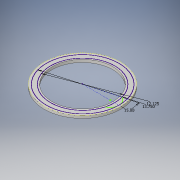
# Autodesk Inventor part: DiskCam
Saved by Autodesk Inventor 2016 (Build 200138000, 138)
## iProperties
Created: 2015-07-20
Part Number: DiskCam
Material: PC/ABS Plastic
Document SubType Name: Modeling
Designer: steele
Density: 0.357273 g/cm^3
Appearance: Smooth - White
Mass: 179.331 g
Surface Area: 1053.95 cm^2
Volume: 501.944 cm^3
Author: steele
Autodesk Inventor part; units mm, degrees
ref_plane "YZ Plane" through (0, 0, 0) normal (1, 0, 0) x (0, 1, 0)
ref_plane "XZ Plane" through (0, 0, 0) normal (0, 1, 0) x (-1, 0, 0)
ref_plane "XY Plane" through (0, 0, 0) normal (0, 0, 1) x (1, 0, 0)
sketch "Sketch1" plane through (0, 0, 0) normal (0, 1, 0) x (-1, 0, 0)
  circle A0 centre (0, 0) radius 146.05
  circle A1 centre (0, 0) radius 184.15
  dimension "camInsideDiameter" = 292.1
  dimension "d1" = 368.3
  constraints: 2 centre point, 2 coincident
  measures "camInsideDiameter" diameter of A0
  measures "d1" diameter of A1
extrude "Extrusion1" add sketch "Sketch1" along normal blind 12.7
sketch "Sketch4" plane through (147.2071, 12.7, 39.444) normal (0.7357, 0, -0.6773) x (0, 1, 0)
  circle A0 centre (0, 0) radius 3.175
  point P0 (-12.7, -128.725)
  dimension "d9" = 6.35
  constraints: 1 centre point
  measures "d9" diameter of A0
sketch "Sketch2" plane through (0, 12.7, 0) normal (0, 1, 0) x (1, 0, 0)
  circle A0 centre (0, 0) radius 146.05 construction
  circle A1 centre (0, 0) radius 184.15 construction
  line L0 (0, 0) -> (147.2071, -39.444) construction
  line L1 (0, 0) -> (184.15, 0) construction
  line L2 (0, 0) -> (147.2071, 39.444) construction
  line L3 (147.2071, -39.444) -> (173.1094, -15.5967)
  line L4 (147.2071, 39.444) -> (173.1094, 15.5967)
  arc A2 (173.1094, -15.5967) -> (173.1094, 15.5967) centre (158.75, 0) ccw
  dimension "oneHalfPhase" = 15
  dimension "d5" = 15
  dimension "innerRadiusForCam" = 152.4
  dimension "innerRadisuForCam" = 152.4
  dimension "d12" = 158.75
  constraints: 10 end point, 2 point on circle, 2 tangent, 1 centre point, 1 horizontal, 1 horizontal alignment, 1 point on line, 1 other
  measures "oneHalfPhase" angle of L0 L1
  measures "d5" angle of L2 L1
  measures "innerRadiusForCam" distance of point (0, 0) L2.end
  measures "innerRadisuForCam" distance of L0.start L0.end
  measures "d12" distance of point (0, 0) A2.centre
sketch "Sketch7" plane through (0, 12.7, 0) normal (0, 1, 0) x (1, 0, 0)
  circle A0 centre (0, 0) radius 153.9875
  circle A1 centre (0, 0) radius 174.625
  line L0 (0, 0) -> (184.15, 0) construction
  circle A2 centre (0, 0) radius 184.15 construction
  line L1 (0, 0) -> (177.8752, 47.6615) construction
  arc A3 (174.625, 0) -> (148.7405, 39.8549) centre (134.2536, 2.1131) ccw
  arc A4 (148.7405, -39.8549) -> (174.625, 0) centre (134.2536, -2.1131) ccw
  dimension "d13" = 349.25
  dimension "d14" = 307.975
  dimension "d15" = 15
  constraints: 6 point on circle, 4 end point, 2 centre point, 2 coincident, 2 point on line, 2 symmetric about line, 1 horizontal, 1 horizontal alignment, 6 other
  measures "d15" angle of L1 L0
equation "\"d5\" = oneHalfPhase"
equation "\"innerRadiusForCam\" = innerRadisuForCam"
body "Solid1"
